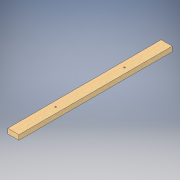
# Autodesk Inventor part: 48in 2x4
Saved by Autodesk Inventor 2017 (Build 210142000, 142)
## iProperties
Created: 2017-05-24
Part Number: 48in 2x4
Material: Pine, Radiata
Document SubType Name: Modeling
Designer: cas7
Density: 0.48 g/cm^3
Appearance: Pine - Coarse
Mass: 1982.18 g
Surface Area: 3164.51 cm^2
Volume: 4129.54 cm^3
Author: cas7
Autodesk Inventor part; units mm, degrees
ref_plane "YZ Plane" through (0, 0, 0) normal (1, 0, 0) x (0, 1, 0)
ref_plane "XZ Plane" through (0, 0, 0) normal (0, 1, 0) x (-1, 0, 0)
ref_plane "XY Plane" through (0, 0, 0) normal (0, 0, 1) x (1, 0, 0)
sketch "Sketch1" plane through (0, 0, 0) normal (0, 0, 1) x (1, 0, 0)
  line L0 (0, 0) -> (0, 38.1)
  line L1 (0, 38.1) -> (88.9, 38.1)
  line L2 (88.9, 38.1) -> (88.9, 0)
  line L3 (88.9, 0) -> (0, 0)
  dimension "d0" = 38.1
  dimension "d1" = 88.9
  constraints: 8 end point, 3 perpendicular, 1 vertical
  measures "d0" distance of L0.start L0.end
  measures "d1" distance of L0.end L1.end
extrude "Extrusion1" add sketch "Sketch1" along normal blind 533.4
sketch "Sketch3" plane through (0, 0, 533.4) normal (0, 0, 1) x (1, 0, 0)
  line L0 (0, 38.1) -> (0, 0) projected
  line L1 (0, 0) -> (88.9, 0) projected
  line L2 (88.9, 0) -> (88.9, 38.1) projected
  line L3 (88.9, 38.1) -> (0, 38.1) projected
extrude "Extrusion2" add sketch "Sketch3" along normal blind 685.8
sketch "Sketch5" plane through (0, 38.1, 0) normal (0, 1, 0) x (1, 0, 0)
  line L0 (0, 0) -> (88.9, 0) projected
  line L1 (0, 0) -> (0, -1219.2) projected
  line L2 (88.9, -1219.2) -> (0, -1219.2) projected
  line L3 (88.9, 0) -> (88.9, -1219.2) projected
  line L4 (88.9, 0) -> (0, 0) projected
  line L5 (88.9, 0) -> (0, 0)
  line L6 (0, -38.1) -> (88.9, -38.1)
  line L7 (0, -295.275) -> (88.9, -295.275)
  line L8 (0, -333.375) -> (88.9, -333.375)
  line L9 (0, -590.55) -> (88.9, -590.55)
  line L10 (0, -628.65) -> (88.9, -628.65)
  line L11 (0, -885.825) -> (88.9, -885.825)
  line L12 (0, -923.925) -> (88.9, -923.925)
  line L13 (0, -1181.1) -> (88.9, -1181.1)
  line L14 (0, -1219.2) -> (88.9, -1219.2)
  dimension "d15" = 38.1
  dimension "d16" = 257.175
  dimension "d17" = 38.1
  dimension "d18" = 257.175
  dimension "d19" = 38.1
  dimension "d20" = 257.175
  dimension "d21" = 38.1
  dimension "d22" = 257.175
  dimension "d23" = 38.1
  constraints: 20 end point, 10 equal length
  measures "d15" distance between parallel lines of L0 L6
  measures "d16" distance between parallel lines of L6 L7
  measures "d17" distance between parallel lines of L7 L8
  measures "d18" distance between parallel lines of L8 L9
  measures "d19" distance between parallel lines of L9 L10
  measures "d20" distance between parallel lines of L10 L11
  measures "d21" distance between parallel lines of L11 L12
  measures "d22" distance between parallel lines of L12 L13
  measures "d23" distance between parallel lines of L13 L14
sketch "Sketch6" plane through (0, 38.1, 0) normal (0, 1, 0) x (1, 0, 0)
  line L0 (88.9, 0) -> (88.9, -336.55)
  line L1 (88.9, -1219.2) -> (88.9, -882.65)
  line L2 (88.9, -1219.2) -> (425.45, -1219.2) construction
  point P0 (44.45, -882.65)
  point P1 (45.955, -336.55)
  dimension "d26" = 90
  constraints: 6 end point, 1 horizontal, 1 perpendicular
  measures "d26" angle of L2 L1
hole "Hole1" at (44.45, 38.1, 882.65) at (45.955, 38.1, 336.55) direction (0, -1, 0) diameter 10.5918 depth 35.179 tip angle 118 thread size "1/2-13 UNC" class "2B" standard "ANSI Unified Screw Threads"
body "Solid1"
